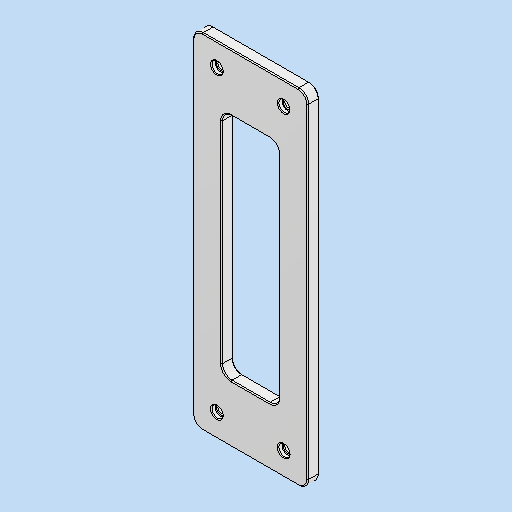
# Autodesk Inventor part: tc-top-bar
Saved by Autodesk Inventor 2026 (Build 300175050, 175E)
## iProperties
Created: 2025-06-05
Part Number: tc-top-bar
Material: ABS Plastic
Document SubType Name: Modeling
Designer: queezz
Density: 1.06 g/cm^3
Appearance: Smooth - White
Author: queezz
Autodesk Inventor part; units mm, degrees
ref_plane "YZ Plane" through (0, 0, 0) normal (1, 0, 0) x (0, 1, 0)
ref_plane "XZ Plane" through (0, 0, 0) normal (0, 1, 0) x (-1, 0, 0)
ref_plane "XY Plane" through (0, 0, 0) normal (0, 0, 1) x (1, 0, 0)
sketch "Sketch1" plane through (0, 0, 0) normal (0, 0, 1) x (1, 0, 0)
  line L0 (-30, 90) -> (30, 90)
  line L1 (30, 90) -> (30, -90)
  line L2 (30, -90) -> (-30, -90)
  line L3 (-30, -90) -> (-30, 90)
  point P0 (0, 0)
  point P1 (30, 0)
  point P2 (0, 90)
  dimension "d0" = 60
  dimension "d1" = 180
  constraints: 8 end point, 2 midpoint, 2 parallel, 1 horizontal, 1 horizontal alignment, 1 perpendicular, 1 vertical alignment
  measures "d0" distance of L0.start L0.end
  measures "d1" distance of L0.end L1.end
extrude "Extrusion1" add sketch "Sketch1" along normal blind 6
sketch "Sketch4" plane through (0, 0, 6) normal (0, 0, 1) x (1, 0, 0)
  line L0 (-15, 60) -> (15, 60)
  line L1 (15, 60) -> (15, -60)
  line L2 (15, -60) -> (-15, -60)
  line L3 (-15, -60) -> (-15, 60)
  line L4 (30, -90) -> (30, 90) projected
  line L5 (30, 90) -> (-30, 90) projected
  point P0 (0, 0)
  point P1 (0, 60)
  point P2 (15, 0)
  dimension "d20" = 15
  dimension "d21" = 30
  constraints: 8 end point, 2 midpoint, 2 parallel, 1 horizontal, 1 horizontal alignment, 1 perpendicular, 1 vertical alignment
  measures "d20" distance between parallel lines of L4 L1
  measures "d21" distance between parallel lines of L0 L5
extrude "Extrusion4" cut sketch "Sketch4" against normal through all
fillet "Fillet1" radius 5 8 edges at (-30, 90, 3) (30, 90, 3) (30, -90, 3) (-30, -90, 3) (-15, 60, 3) (15, 60, 3) (15, -60, 3) (-15, -60, 3)
chamfer "Chamfer2" distance 0.5 angle 45 32 edges at (0, 90, 6) (-28.5355, 88.5355, 6) (-30, 0, 6) (-28.5355, -88.5355, 6) (0, -90, 6) (28.5355, -88.5355, 6) (30, 0, 6) (28.5355, 88.5355, 6) (0, 90, 0) (-28.5355, 88.5355, 0) (-30, 0, 0) (-28.5355, -88.5355, 0) (0, -90, 0) (28.5355, -88.5355, 0) (30, 0, 0) (28.5355, 88.5355, 0) (-15, 0, 6) (-13.5355, 58.5355, 6) (0, 60, 6) (13.5355, 58.5355, 6) (15, 0, 6) (13.5355, -58.5355, 6) (0, -60, 6) (-13.5355, -58.5355, 6) (-15, 0, 0) (-13.5355, -58.5355, 0) (0, -60, 0) (13.5355, -58.5355, 0) (15, 0, 0) (13.5355, 58.5355, 0) (0, 60, 0) (-13.5355, 58.5355, 0)
sketch "Sketch5" plane through (0, 0, 6) normal (0, 0, 1) x (1, 0, 0)
  line L0 (-17.5, 78) -> (17.5, 78) construction
  line L1 (17.5, 78) -> (17.5, -78) construction
  line L2 (17.5, -78) -> (-17.5, -78) construction
  line L3 (-17.5, -78) -> (-17.5, 78) construction
  line L4 (25, 90) -> (-25, 90) construction
  point P0 (0, 0)
  point P1 (0, 78)
  point P2 (17.5, 0)
  point P3 (81.7088, -86.6952)
  dimension "d24" = 12
  dimension "d25" = 35
  constraints: 8 end point, 4 coincident, 2 midpoint, 2 parallel, 1 horizontal, 1 horizontal alignment, 1 perpendicular, 1 vertical alignment
  measures "d24" distance between parallel lines of L4 L0
  measures "d25" distance of L0.start L0.end
hole "Hole1" at (-17.5, 78, 6) at (17.5, 78, 6) at (17.5, -78, 6) at (-17.5, -78, 6) at (81.7088, -86.6952, 6) direction (0, 0, -1) diameter 3.6 end through all counterbore diameter 5.8 counterbore depth 2
chamfer "Chamfer3" distance 0.4 angle 45 12 edges at (17.5, -76.2, 0) (-17.5, -76.2, 0) (-17.5, 79.8, 0) (17.5, 79.8, 0) (17.5, 80.9, 6) (-17.5, 80.9, 6) (17.5, 79.8, 4) (-17.5, 79.8, 4) (-17.5, -75.1, 6) (-17.5, -76.2, 4) (17.5, -76.2, 4) (17.5, -75.1, 6)
equation "\"d0\" = width"
equation "\"d1\" = hight"
equation "\"width\" = 60"
equation "\"hight\" = 180"
body "Solid1"
